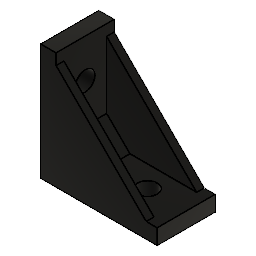
2020_Corner_Bracket_F01 (Autodesk Fusion 360 design; units mm, degrees)
Autodesk Fusion 360 part; units mm, degrees
sketch "スケッチ1" plane through (0, 0, 0) normal (0, 1, 0) x (1, 0, 0)
  line L0 (0, 0) -> (0, -30)
  line L1 (0, -30) -> (4, -30)
  line L2 (4, -30) -> (4, -4)
  line L3 (4, -27.1719) -> (27.1719, -4)
  line L4 (4, -4) -> (30, -4)
  line L5 (30, -4) -> (30, 0)
  line L6 (30, 0) -> (0, 0)
  dimension "d1" = 30
  dimension "d2" = 30
  dimension "d3" = 4
  dimension "d4" = 4
  dimension "d5" = 32.77
  dimension "d6" = 45
  measures "d3" distance of L0.start
  measures "d4" distance of L0.start
  measures "d6" angle of L3 L4
extrude "押し出し1" add sketch "スケッチ1" along normal mid plane 15
extrude "押し出し2" cut sketch "スケッチ1" along normal mid plane 11 contours L2 L3 L4
chamfer "面取り1" distance 6 angle 45 1 edges at (4, 0, 4)
hole "穴1" at (20, 0, 4) direction (0, 0, -1) diameter 5 depth 4 tip angle 118
hole "穴2" at (4, 0, 20) direction (-1, 0, 0) diameter 5 depth 4 tip angle 118
